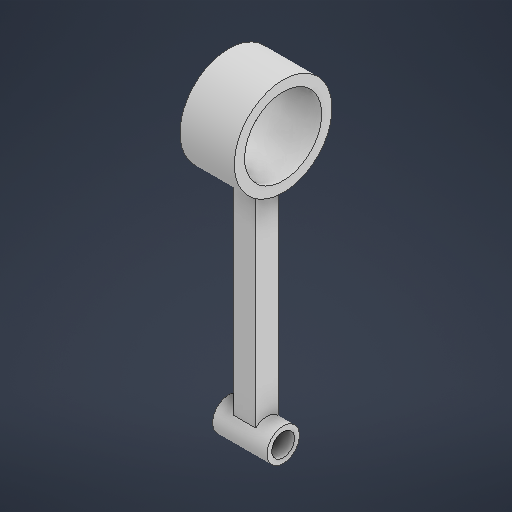
# Autodesk Inventor part: guide
Saved by Autodesk Inventor 2026.1 (Build 301233020, 233B)
## iProperties
Created: 2025-12-31
Part Number: guide
Material: Generic
Document SubType Name: Modeling
Designer: Austin Ngobeni
Density: 1 g/cm^3
Appearance: Default
Author: Austin Ngobeni
Autodesk Inventor part; units mm, degrees
ref_plane "YZ Plane" through (0, 0, 0) normal (1, 0, 0) x (0, 1, 0)
ref_plane "XZ Plane" through (0, 0, 0) normal (0, 1, 0) x (-1, 0, 0)
ref_plane "XY Plane" through (0, 0, 0) normal (0, 0, 1) x (1, 0, 0)
sketch "Sketch1" plane through (0, 0, 0) normal (1, 0, 0) x (0, 1, 0)
  circle A0 centre (0, 0) radius 5.25
  line L0 (0, 0) -> (16.2396, 0) construction
  line L1 (5.4642, 5.1373) -> (101.0943, 5.1373)
  line L2 (5.4642, -5.1373) -> (101.0943, -5.1373)
  circle A1 centre (123, 0) radius 22.5
  circle A2 centre (123, 0) radius 17.75
  circle A3 centre (0, 0) radius 7.5
  dimension "d20" = 15
  dimension "d0" = 10.5
  dimension "d14" = 45
  dimension "d16" = 35.5
  dimension "d17" = 123
  constraints: 6 end point, 4 coincident, 3 centre point, 2 horizontal, 2 point on circle, 1 horizontal alignment, 1 symmetric about line, 3 other
  measures "d0" diameter of A0
  measures "d14" diameter of A1
  measures "d16" diameter of A2
  measures "d17" distance of point (0, 0) A1.centre
extrude "Extrusion1" add sketch "Sketch1" along normal mid plane 25 contours A3 | A1
extrude "Extrusion2" add sketch "Sketch1" along normal mid plane 10 contours L1 A1 L2 A3
body "Solid1"
